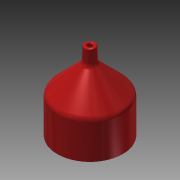
# Autodesk Inventor part: vacuum-resivoir
Saved by Autodesk Inventor 2015 (Build 190159000, 159)
## iProperties
Created: 2015-12-02
Part Number: vacuum-resivoir
Material: Generic
Document SubType Name: Modeling
Designer: caleb
Density: 1 g/cm^3
Appearance: Default
Author: caleb
Autodesk Inventor part; units mm, degrees
ref_plane "YZ Plane" through (0, 0, 0) normal (1, 0, 0) x (0, 1, 0)
ref_plane "XZ Plane" through (0, 0, 0) normal (0, 1, 0) x (-1, 0, 0)
ref_plane "XY Plane" through (0, 0, 0) normal (0, 0, 1) x (1, 0, 0)
sketch "Sketch2" plane through (0, 0, 0) normal (0, 1, 0) x (-1, 0, 0)
  line L0 (15.5, 0) -> (15.5, 17.3284)
  line L1 (15.5, 17.3284) -> (2.7, 30.1284)
  line L2 (2.7, 30.1284) -> (2.55, 37.1284)
  line L3 (2.55, 37.1284) -> (1.15, 37.1284)
  line L4 (1.15, 37.1284) -> (1.15, 28.85)
  line L5 (1.15, 28.85) -> (12.5, 17.5)
  line L6 (12.5, 17.5) -> (12.5, 0)
  line L7 (12.5, 0) -> (15.5, 0)
  line L8 (0, -7.4257) -> (0, 44.5541) projected
  point P0 (0, 0)
  dimension "d5" = 12.5
  dimension "d6" = 17.5
  dimension "d7" = 3
  dimension "d8" = 2
  dimension "d9" = 1.4
  dimension "d10" = 2.55
  dimension "d11" = 2.7
  dimension "d12" = 7
  dimension "d13" = 135
  constraints: 17 end point, 3 perpendicular, 2 parallel, 1 horizontal alignment, 1 vertical
  measures "d5" distance from line of point (0, 0) L6
  measures "d6" distance of L5.end L6.end
  measures "d7" distance of L6.end L0.start
  measures "d8" distance between parallel lines of L1 L5
  measures "d9" distance of L2.end L3.end
  measures "d10" horizontal distance of point (0, 0) L2.end
  measures "d11" horizontal distance of point (0, 0) L1.end
  measures "d12" vertical distance of L2.end L1.end
  measures "d13" angle of L6 L5
revolve "Revolution1" add sketch "Sketch2" angle 360 about axis through (0, 0, -10) along (0, 0, 1)
fillet "Fillet1" radius 0.5 2 edges at (2.55, 0, 37.1284) (1.15, 0, 37.1284)
fillet "Fillet2" radius 3 4 edges at (15.5, 0, 17.3284) (2.7, 0, 30.1284) (12.5, 0, 17.5) (1.15, 0, 28.85)
body "Solid2"
